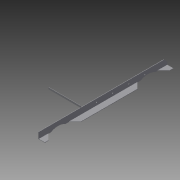
# Autodesk Inventor part: Conveyor Support
Saved by Autodesk Inventor 2015 (Build 190159000, 159)
## iProperties
Created: 2015-01-17
Part Number: Conveyor Support
Material: Generic
Document SubType Name: Modeling
Designer: chapale16
Density: 1 g/cm^3
Appearance: Default
Author: chapale16
Autodesk Inventor part; units mm, degrees
ref_plane "YZ Plane" through (0, 0, 0) normal (1, 0, 0) x (0, 1, 0)
ref_plane "XZ Plane" through (0, 0, 0) normal (0, 1, 0) x (-1, 0, 0)
ref_plane "XY Plane" through (0, 0, 0) normal (0, 0, 1) x (1, 0, 0)
sketch "Sketch1" plane through (0, 0, 0) normal (0, 0, 1) x (1, 0, 0)
  line L0 (0, 0) -> (0, 50.8)
  line L1 (0, 0) -> (50.8, 0)
  line L2 (3.175, 50.8) -> (3.175, 3.175)
  line L3 (3.175, 3.175) -> (50.8, 3.175)
  line L4 (0, 50.8) -> (3.175, 50.8)
  line L5 (50.8, 3.175) -> (50.8, 0)
  dimension "d0" = 50.8
  dimension "d1" = 50.8
  dimension "d2" = 3.175
  constraints: 12 end point, 2 horizontal, 1 perpendicular, 1 vertical, 1 other
  measures "d0" distance of L0.start L0.end
  measures "d1" distance of L0.start L1.end
  measures "d2" distance between parallel lines of L0 L2
extrude "Extrusion1" add sketch "Sketch1" along normal blind 1016
sketch "Sketch2" plane through (3.175, 3.175, 0) normal (0, 1, 0) x (1, 0, 0)
  line L0 (-3.175, 0) -> (-3.175, -1016) projected
  line L1 (47.625, -1016) -> (-3.175, -1016)
  line L2 (-3.175, -1016) -> (-3.175, -990.6)
  line L3 (-3.175, -990.6) -> (47.625, -990.6)
  line L4 (47.625, -990.6) -> (47.625, -1016)
  line L5 (0, 0) -> (0, -1016) projected
  line L6 (47.625, 0) -> (47.625, -1016) projected
  line L7 (0, -990.6) -> (47.625, -990.6)
  line L8 (47.625, -990.6) -> (47.625, -830.58)
  line L9 (47.625, -830.58) -> (0, -830.58)
  line L10 (0, -830.58) -> (0, -990.6)
  line L11 (47.625, 0) -> (0, 0)
  line L12 (0, 0) -> (0, -25.4)
  line L13 (0, -25.4) -> (47.625, -25.4)
  line L14 (47.625, -25.4) -> (47.625, 0)
  line L15 (47.625, -25.4) -> (0, -25.4)
  line L16 (0, -25.4) -> (0, -185.42)
  line L17 (0, -185.42) -> (47.625, -185.42)
  line L18 (47.625, -185.42) -> (47.625, -25.4)
  dimension "d5" = 25.4
  dimension "d6" = 160.02
  dimension "d7" = 25.4
  dimension "d8" = 160.02
  constraints: 32 end point, 8 parallel, 6 point on line, 4 horizontal, 4 perpendicular
  measures "d5" distance of L1.end L2.end
  measures "d6" distance of L8.end L7.end
  measures "d7" distance of L12.end L11.end
  measures "d8" distance of L16.end L15.end
extrude "Extrusion2" cut sketch "Sketch2" against normal blind 1016 contours L5 L9 L6 L3 | L5 L13 L6 L17
sketch "Sketch5" plane through (3.175, 3.175, 185.42) normal (0, 1, 0) x (1, 0, 0)
  line L0 (47.625, 0) -> (47.625, -645.16) projected
  line L1 (0, 0) -> (47.625, 0)
  line L2 (47.625, 0) -> (47.625, -50.8)
  line L3 (47.625, -50.8) -> (0, -50.8)
  line L4 (0, -50.8) -> (0, 0)
  line L5 (0, 0) -> (0, -645.16) projected
  line L6 (47.625, -645.16) -> (0, -645.16)
  line L7 (0, -645.16) -> (0, -594.36)
  line L8 (0, -594.36) -> (47.625, -594.36)
  line L9 (47.625, -594.36) -> (47.625, -645.16)
  point P0 (-3.175, 185.42)
  dimension "d21" = 50.8
  dimension "d22" = 50.8
  constraints: 16 end point, 4 parallel, 2 horizontal, 2 perpendicular, 2 point on line
  measures "d21" distance of L1.end L2.end
  measures "d22" distance of L6.end L7.end
extrude "Extrusion4" cut sketch "Sketch5" against normal blind 1016 contours L0 L3 L4 L1 | L0 L6 L5 L8
sketch "Sketch6" plane through (3.175, 3.175, 0) normal (1, 0, 0) x (0, 0, -1)
  circle A0 centre (-152.4, -101.6) radius 114.3
  circle A1 centre (-863.6, -101.6) radius 114.3
  point P0 (0, -3.175)
  dimension "d25" = 228.6
  constraints: 2 centre point, 2 coincident
  measures "d25" diameter of A0
extrude "Extrusion5" cut sketch "Sketch6" against normal blind 1016
sketch "Sketch7" plane through (3.175, 3.175, 1016) normal (0, 1, 0) x (1, 0, 0)
  line L0 (0, 990.6) -> (0, 921.712) projected
  line L1 (47.625, 990.6) -> (0, 990.6)
  line L2 (0, 990.6) -> (0, 939.8)
  line L3 (0, 939.8) -> (47.625, 939.8)
  line L4 (47.625, 939.8) -> (47.625, 990.6)
  line L5 (0, 94.288) -> (0, 25.4) projected
  line L6 (47.625, 24.8924) -> (0, 24.8924)
  line L7 (0, 24.8924) -> (0, 75.6924)
  line L8 (0, 75.6924) -> (47.625, 75.6924)
  line L9 (47.625, 75.6924) -> (47.625, 24.8924)
  point P0 (-3.175, 1016)
  dimension "d28" = 50.8
  dimension "d29" = 50.8
  constraints: 16 end point, 4 parallel, 3 point on line, 2 horizontal, 2 perpendicular
  measures "d28" distance of L2.end L1.end
  measures "d29" distance of L6.end L7.end
extrude "Extrusion6" add sketch "Sketch7" against normal blind 3.175
sketch "Sketch8" plane through (3.175, 3.175, 0) normal (1, 0, 0) x (0, 0, -1)
  line L0 (0, 47.625) -> (-1016, 47.625) projected
  line L1 (-26.088, 47.625) -> (2.2813, 19.2557)
  line L2 (-26.088, 47.625) -> (14.0323, 47.625) construction
  line L3 (2.2813, 19.2557) -> (0, 47.625)
  line L4 (0, 47.625) -> (-26.088, 47.625)
  point P0 (0, -3.175)
  dimension "d32" = 45
  constraints: 8 end point, 3 point on line, 1 equal length, 1 horizontal
  measures "d32" angle of L1 L2
extrude "Extrusion7" cut sketch "Sketch8" against normal blind 3.175
sketch "Sketch9" plane through (3.175, 3.175, 1016) normal (1, 0, 0) x (0, 0, -1)
  line L0 (989.912, 47.625) -> (0, 47.625) projected
  line L1 (330.2, 47.625) -> (330.2, -3.175)
  point P0 (1016, -3.175)
  point P1 (330.2, 23.8125)
  point P2 (838.2, 22.225)
  point P3 (711.2, 22.225)
  point P4 (584.2, 22.225)
  point P5 (457.2, 22.225)
  constraints: 2 end point, 1 point on line, 1 vertical
hole "Hole2" at (3.175, 25.4, 177.8) at (3.175, 25.4, 304.8) at (3.175, 25.4, 431.8) at (3.175, 25.4, 558.8) direction (-1, 0, 0) diameter 9.525 end through all
sketch "Sketch10" plane through (3.175, 3.175, 1016) normal (0, 1, 0) x (1, 0, 0)
  line L0 (0, 75.6924) -> (43.0144, 32.678)
  line L1 (0, 75.6924) -> (60.8315, 75.6924) construction
  line L2 (43.0144, 32.678) -> (47.625, 28.0674)
  line L3 (47.625, 75.6924) -> (47.625, 0) projected
  line L4 (47.625, 75.6924) -> (0, 75.6924)
  line L5 (0, 94.288) -> (0, 75.6924) projected
  line L6 (0, 236.22) -> (70.4888, 306.7088)
  line L7 (0, 236.22) -> (99.6862, 236.22) construction
  line L8 (70.4888, 306.7088) -> (70.4888, 236.22)
  line L9 (70.4888, 236.22) -> (0, 236.22)
  line L10 (0, 779.78) -> (0, 236.22) projected
  line L11 (0, 779.78) -> (47.625, 732.155)
  line L12 (47.625, 732.155) -> (47.625, 779.78)
  line L13 (47.625, 779.78) -> (47.625, 236.22) projected
  line L14 (47.625, 779.78) -> (0, 779.78)
  line L15 (0, 939.8) -> (47.625, 987.425)
  line L16 (47.625, 1016) -> (47.625, 939.8) projected
  line L17 (47.625, 939.8) -> (0, 939.8)
  point P0 (-3.175, 1016)
  dimension "d42" = 45
  dimension "d43" = 45
  constraints: 26 end point, 6 perpendicular, 3 point on line, 2 equal length, 2 horizontal, 1 collinear
  measures "d42" angle of L0 L1
  measures "d43" angle of L7 L6
extrude "Extrusion8" cut sketch "Sketch10" against normal blind 25.4 contours L4 L3 L2 L0 | L6 L13 L9 | L6 L8 L9 L13 | L14 L12 L11 | L15 L16 L17
sketch "Sketch11" plane through (3.175, 3.175, 1016) normal (1, 0, 0) x (0, 0, -1)
  line L0 (989.912, 47.625) -> (0, 47.625) projected
  line L1 (330.2, 47.625) -> (332.5489, 47.625)
  line L2 (332.5489, 47.625) -> (332.5489, 61.5215)
  line L3 (332.5489, 61.5215) -> (330.2, 61.5215)
  line L4 (330.2, 61.5215) -> (330.2, 47.625)
  point P0 (1016, -3.175)
  constraints: 8 end point, 2 parallel, 1 horizontal, 1 perpendicular, 1 point on line
extrude "Extrusion9" add sketch "Sketch11" against normal blind 254
body "Solid1"
